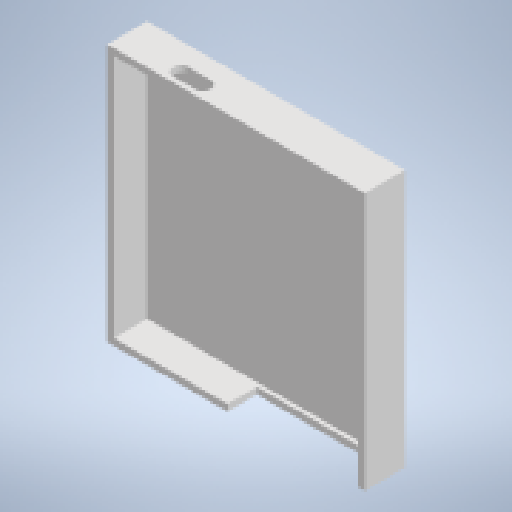
# Autodesk Inventor part: Base REV 1.0
Saved by Autodesk Inventor 2024 (Build 280153000, 153)
## iProperties
Created: 2025-07-25
Part Number: Base REV 1.0
Material: Generic
Document SubType Name: Modeling
Designer: Gavin
Density: 1 g/cm^3
Appearance: Default
Author: Gavin
Autodesk Inventor part; units mm, degrees
ref_plane "YZ Plane" through (0, 0, 0) normal (1, 0, 0) x (0, 1, 0)
ref_plane "XZ Plane" through (0, 0, 0) normal (0, 1, 0) x (-1, 0, 0)
ref_plane "XY Plane" through (0, 0, 0) normal (0, 0, 1) x (1, 0, 0)
sketch "Sketch1" plane through (0, 0, 0) normal (0, 0, 1) x (1, 0, 0)
  line L0 (100.75, -55.25) -> (169.75, -55.25)
  line L1 (169.75, -55.25) -> (169.75, -124.25)
  line L2 (169.75, -124.25) -> (100.75, -124.25)
  line L3 (100.75, -124.25) -> (100.75, -55.25)
  line L4 (167.75, -122.25) -> (102.75, -122.25) projected
  line L5 (167.75, -57.25) -> (167.75, -122.25) projected
  line L6 (102.75, -57.25) -> (167.75, -57.25) projected
  line L7 (102.75, -122.25) -> (102.75, -57.25) projected
  point P0 (0, 0)
  dimension "d0" = 69
  dimension "d1" = 69
  dimension "d2" = 2
  dimension "d3" = 2
  constraints: 8 end point, 2 parallel, 1 horizontal, 1 perpendicular
  measures "d0" distance of L1.end L2.end
  measures "d1" distance of L0.end L1.end
  measures "d2" distance between parallel lines of L4 L2
  measures "d3" distance between parallel lines of L1 L5
extrude "Base Shell Extrusion" add sketch "Sketch1" along normal blind 5.25 and the other way blind 5.5 contours L0 L1 L2 L3 | L4 L7 L6 L5
shell "Shell1" thickness 1.75 removed faces 1 at (123.75, -101.25, 5.25)
sketch "USB C Port hole sketch" plane through (100.75, -55.25, 5.25) normal (0, 1, 0) x (1, 0, 0)
  line L0 (19.22, 1.905) -> (22.41, 1.905) projected
  arc A0 (22.41, 1.905) -> (23.69, 3.185) centre (22.41, 3.185) ccw projected
  line L1 (23.69, 3.185) -> (23.69, 3.785) projected
  arc A1 (23.69, 3.785) -> (22.41, 5.065) centre (22.41, 3.785) ccw projected
  line L2 (22.41, 5.065) -> (19.22, 5.065) projected
  line L3 (16.03, 5.065) -> (19.22, 5.065) projected
  arc A2 (16.03, 5.065) -> (14.75, 3.785) centre (16.03, 3.785) ccw projected
  line L4 (14.75, 3.185) -> (14.75, 3.785) projected
  arc A3 (14.75, 3.185) -> (16.03, 1.905) centre (16.03, 3.185) ccw projected
  line L5 (19.22, 1.905) -> (16.03, 1.905) projected
  arc A4 (22.41, 1.905) -> (23.69, 3.185) centre (22.41, 3.185) ccw
  arc A5 (14.75, 3.185) -> (16.03, 1.905) centre (16.03, 3.185) ccw
  arc A6 (16.03, 5.065) -> (14.75, 3.785) centre (16.03, 3.785) ccw
  arc A7 (23.69, 3.785) -> (22.41, 5.065) centre (22.41, 3.785) ccw
  line L6 (14.75, 3.785) -> (14.75, 3.185)
  line L7 (16.03, 5.065) -> (22.41, 5.065)
  line L8 (23.69, 3.785) -> (23.69, 3.185)
  line L9 (16.03, 1.905) -> (22.41, 1.905)
  line L10 (22.41, 1.405) -> (19.22, 1.405)
  line L11 (19.22, 1.405) -> (16.03, 1.405)
  arc A8 (14.25, 3.185) -> (16.03, 1.405) centre (16.03, 3.185) ccw
  line L12 (14.25, 3.185) -> (14.25, 3.785)
  arc A9 (16.03, 5.565) -> (14.25, 3.785) centre (16.03, 3.785) ccw
  line L13 (16.03, 5.565) -> (19.22, 5.565)
  line L14 (19.22, 5.565) -> (22.41, 5.565)
  arc A10 (24.19, 3.785) -> (22.41, 5.565) centre (22.41, 3.785) ccw
  line L15 (24.19, 3.785) -> (24.19, 3.185)
  arc A11 (22.41, 1.405) -> (24.19, 3.185) centre (22.41, 3.185) ccw
  point P0 (-100.75, 5.25)
  dimension "d24" = 0.5
  constraints: 20 end point, 19 point on circle, 8 centre point, 5 tangent, 4 coincident, 3 collinear, 2 concentric, 1 perpendicular, 9 other
  measures "d24" distance between parallel lines of L0 L10
sketch "Rough encoder hole" plane through (100.75, -124.25, 5.25) normal (0, -1, 0) x (1, 0, 0)
  line L0 (67.25, -7.8767) -> (32.25, -7.8767)
  line L1 (32.25, -7.8767) -> (32.25, 0.1233)
  line L2 (32.25, 0.1233) -> (67.25, 0.1233)
  line L3 (67.25, 0.1233) -> (67.25, -7.8767)
  line L4 (67.25, -9) -> (67.25, 0) projected
  point P0 (-100.75, -5.25)
  dimension "d13" = 35
  dimension "d14" = 8
  dimension "d17" = 0
  constraints: 8 end point, 2 parallel, 1 horizontal, 1 perpendicular
  measures "d13" distance of L1.end L2.end
  measures "d14" distance of L0.end L1.end
  measures "d17" distance between parallel lines of L4 L3
extrude "Rough Encoder Hole Extrusion" cut sketch "Rough encoder hole" against normal up to surface (1.75 mm away)
extrude "USB C Hole Extrusion" cut sketch "USB C Port hole sketch" against normal up to surface (1.75 mm away) contours L5 A3 L4 A2 L3 L2 A1 L1 A0 L0 | L10 L11 A8 L12 A9 L13 L14 A10 L15 A11
